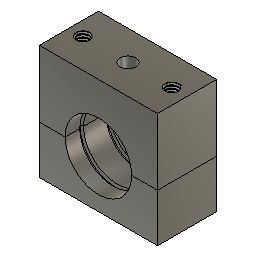
2-Part Thunderhex Bearing Mount (Autodesk Fusion 360 design; units mm, degrees)
Autodesk Fusion 360 part; units mm, degrees
note: some values were not read from the file. Chosen so that the rebuilt part matches the saved one: which face or edge a step refers to; a direction; where a thread starts. Set by a fixed rule: which sketch regions a step uses.
sketch "Sketch1" plane through (0, 0, 0) normal (0, 1, 0) x (1, 0, 0)
  circle A0 centre (0, 0) radius 14.2875
  line L0 (-25.4, 0) -> (25.4, 0)
  line L1 (25.4, 0) -> (25.4, -28.575)
  line L2 (25.4, -28.575) -> (-25.4, -28.575)
  line L3 (-25.4, -28.575) -> (-25.4, 0)
  line L4 (0, 0) -> (0, -28.575) construction
  line L5 (-25.4, -14.2875) -> (25.4, -14.2875)
  line L6 (25.4, 0) -> (25.4, 20.6375)
  line L7 (25.4, 20.6375) -> (-25.4, 20.6375)
  line L8 (-25.4, 20.6375) -> (-25.4, 0)
  line L9 (25.4, 14.2875) -> (-25.4, 14.2875) construction
  circle A1 centre (0, 0) radius 11.1125
  line L10 (-3.6021, -10.5125) -> (3.6021, -10.5125)
  line L11 (25.4, -11.1125) -> (-25.4, -11.1125) construction
  circle A2 centre (0, 0) radius 15.875
  dimension "d1" = 28.575
  dimension "d2" = 50.8
  dimension "d3" = 28.575
  dimension "d30" = 6.35
  dimension "d31" = 3.175
  dimension "d36" = 0.6
  dimension "d37" = 31.75
  constraint coincident A0.centre L4.start
  constraint horizontal L0
  constraint vertical L1
  constraint horizontal L2
  constraint vertical L3
  constraint coincident A0.centre L0
  constraint coincident L2 L4.end
  constraint perpendicular L2 L4
  constraint symmetric L1 L3 L4
  constraint coincident L3 L5.start
  constraint coincident L1 L5.end
  constraint perpendicular L1 L5
  constraint tangent A0 L5
  constraint perpendicular L0 L6
  constraint perpendicular L3 L7
  constraint perpendicular L0 L8
  constraint coincident L6 L9.start
  constraint coincident L8 L9.end
  constraint perpendicular L8 L9
  constraint tangent A0 L9
  constraint coincident A1 L10.start
  constraint coincident A1 L10.end
  constraint parallel L0 L10
  constraint coincident L1 L11.start
  constraint coincident L3 L11.end
  constraint perpendicular L3 L11
  constraint tangent A1 L11
  constraint concentric A1 A2
  measures "d1" diameter of A0
  measures "d2" distance of L0.start L0.end
  measures "d3" distance of L0.end L1.end
  measures "d30" distance of L7 L9
  measures "d31" distance of A0 A1
  measures "d36" distance of L10 L11
  measures "d37" diameter of A2
extrude "Extrude1" add sketch "Sketch1" along normal blind 25.4 contours L5 A2 | L1 L2 L3 L5 A2 makes body 1
sketch "Sketch2" plane through (0, 0, 14.2875) normal (0, 0, -1) x (1, 0, 0)
  line L0 (25.4, 0) -> (-25.4, 0) construction
  line L1 (-25.4, 0) -> (-25.4, -25.4) construction
  line L2 (-25.4, -25.4) -> (25.4, -25.4) construction
  line L3 (25.4, -25.4) -> (25.4, 0) construction
  line L4 (0, -25.4) -> (0, 0) construction
  line L5 (-25.4, -12.7) -> (25.4, -12.7) construction
  point P0 (0, -12.7)
  point P1 (-19.05, -12.7)
  point P2 (19.05, -12.7)
  dimension "d6" = 6.35
  constraint midpoint L2 L4.start
  constraint coincident L4.end origin
  constraint midpoint L1 L5.start
  constraint midpoint L3 L5.end
  constraint midpoint L5 P0
  constraint coincident L5 P1
  constraint symmetric L4 P1 P2
  measures "d6" distance of L1 P1
hole "Hole1" at (0, 12.7, 14.2875) direction (0, 0, 1) diameter 6.7564 depth 22.86 tip angle 180 counterbore diameter 11.1252 counterbore depth 6.35 bodies 1
move_face "OffsetFaces1" offset -1.27 1 faces at (0.2764, 17.5138, 20.6375) on bodies 1
extrude "Extrude2" add sketch "Sketch1" along normal up to surface (25.4 mm away) contours A0 L0 L5 A2 | A0 L0 L5 A2 | L0 L1 L5 A2 | L0 L3 L5 A2 bodies 1
hole "Hole2" at (0, 12.7, 14.2875) direction (0, 0, -1) diameter 6.7564 depth 14.3002 tip angle 180 counterbore diameter 11.1252 counterbore depth 6.35 bodies 1
extrude "Extrude3" add sketch "Sketch1" along normal up to surface (25.4 mm away) separate body contours A0 L0 A2 | L0 L6 L7 L8 A2 makes body 2
extrude "Extrude5" cut sketch "Sketch1" along normal blind 1.651 from surface at 17.4625 contours A0 L0 L5 A2 | A0 L0 A2 | A0 L0 L5 A2 | L5 A2 bodies 1 2
extrude "Extrude6" cut sketch "Sketch1" against normal blind 1.651 from surface at 7.9375 contours A0 L0 L5 A2 | A0 L0 A2 | A0 L0 L5 A2 | L5 A2 bodies 1 2
sketch "Sketch3" plane through (0, 0, -20.6375) normal (0, 0, -1) x (1, 0, 0)
  line L0 (-25.4, -25.4) -> (25.4, -25.4)
  line L1 (25.4, -25.4) -> (25.4, 0)
  line L2 (25.4, 0) -> (-25.4, 0)
  line L3 (-25.4, 0) -> (-25.4, -25.4)
  line L4 (-25.4, -25.4) -> (25.4, -25.4)
  line L5 (25.4, -25.4) -> (25.4, 0)
  line L6 (25.4, 0) -> (-25.4, 0)
  line L7 (-25.4, 0) -> (-25.4, -25.4)
  point P0 (-19.05, -12.7)
  point P1 (19.05, -12.7)
hole "Hole3" at (-19.05, 12.7, -20.6375) at (19.05, 12.7, -20.6375) direction (0, 0, 1) diameter 7.1374 depth 20.6375 tip angle 180 bodies 2
hole "Hole4" at (-19.05, 12.7, -20.6375) at (19.05, 12.7, -20.6375) direction (0, 0, 1) diameter 5.1308 depth 63.5 tip angle 180 bodies 1
thread "Thread1" "ANSI Unified Screw Threads 0.25 1/4-20 UNC 1B" major diameter 6.35 minor diameter 5.1181 pitch 1.27 angle 60 modelled right hand crest width 0.3461 on face at (19.1779, 15.2622, 9.525) crest through (19.05, 15.259, 0.9525) on face at (-18.9221, 15.2622, 9.525) crest through (-19.05, 15.259, 0.9525) on bodies 1
